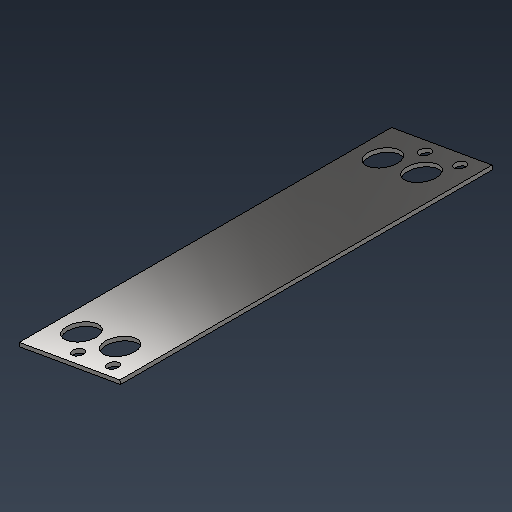
# Autodesk Inventor part: SteelFront
Saved by Autodesk Inventor 2026.2 (Build 302298010, 298A)
## iProperties
Created: 2026-04-07
Part Number: SteelFront
Material: Steel, Alloy
Document SubType Name: Modeling
Designer: szymo
Density: 7.73 g/cm^3
Appearance: Semi-Polished(2)
Mass: 19.4408 g
Surface Area: 54.2307 cm^2
Volume: 2.51498 cm^3
Author: szymo
Autodesk Inventor part; units mm, degrees
ref_plane "YZ Plane" through (0, 0, 0) normal (1, 0, 0) x (0, 1, 0)
ref_plane "XZ Plane" through (0, 0, 0) normal (0, 1, 0) x (-1, 0, 0)
ref_plane "XY Plane" through (0, 0, 0) normal (0, 0, 1) x (1, 0, 0)
sketch "Sketch1" plane through (0, 0, 0) normal (0, 0, 1) x (1, 0, 0)
  line L0 (0, -95.5) -> (0, -82.632) construction
  line L1 (2, -82.632) -> (2, -91.5) construction
  line L2 (2, -91.5) -> (4, -91.5) construction
  line L3 (4, -91.5) -> (0, -95.5) construction
  circle A0 centre (14.5, -55.2958) radius 14.5 construction
  line L4 (2.3736, -91.3) -> (29.4, -86.5356)
  line L5 (29.4, -86.5356) -> (29.2264, -85.5508)
  line L6 (29.2264, -85.5508) -> (2.2, -90.3152)
  line L7 (2.2, -90.3152) -> (2.3736, -91.3)
  line L8 (29.4, -86.5356) -> (29.4, -70.3377) construction
  line L9 (25, -86.2958) -> (4.5, -86.2958) projected
  line L10 (4.5, -86.2958) -> (4.5, -69.7958) projected
  line L11 (25, -69.7958) -> (4.5, -69.7958) projected
  line L12 (25, -86.2958) -> (25, -69.7958) projected
  line L13 (0, -82.632) -> (2, -82.632) projected
  dimension "d0" = 1
  dimension "d1" = 0.2
  dimension "d2" = 0.2
  dimension "d3" = 0.4
  dimension "d4" = 0
  constraints: 10 end point, 2 parallel, 1 perpendicular, 1 vertical
  measures "d0" distance between parallel lines of L6 L4
  measures "d1" distance from line of L1 L6.end
  measures "d2" distance from line of L2 L4.start
  measures "d3" distance edge to line of A0 L8
  measures "d4" distance from line of L6 L9.start
extrude "Extrusion1" add sketch "Sketch1" along normal mid plane 100 contours L7 L6 L5 L4
sketch "Sketch2" plane through (29.4, -86.5356, -50) normal (0.17361, -0.9848145, 0) x (0.9848145, 0.17361, 0)
  line L0 (-25.6154, 16.5) -> (-25.6154, 83.5) projected
  line L1 (-27.6462, 0) -> (-27.6462, 1) projected
  circle A0 centre (-5.2783, 96.6469) radius 1.5
  circle A1 centre (-14.8697, 96.6469) radius 1.5
  circle A2 centre (-14.8697, 3.3531) radius 1.5
  circle A3 centre (-5.2783, 3.3531) radius 1.5
  circle A4 centre (-9.5918, 90.5) radius 4
  circle A5 centre (-20.1476, 90.5) radius 4
  circle A6 centre (-9.5918, 9.5) radius 4
  circle A7 centre (-20.1476, 9.5) radius 4
  line L2 (-27.6462, 99) -> (-27.0065, 99) projected
  line L3 (-27.0065, 99) -> (-27.0065, 82.5) projected
  line L4 (-27.0065, 82.5) -> (-27.6462, 82.5) projected
  line L5 (-27.6462, 17.5) -> (-27.6462, 82.5) projected
  line L6 (-27.6462, 17.5) -> (-27.0065, 17.5) projected
  line L7 (-27.0065, 17.5) -> (-27.0065, 1) projected
  line L8 (-27.0065, 1) -> (-27.6462, 1) projected
  line L9 (-2.2607, 0) -> (-27.6462, 0) projected
  line L10 (-2.2607, 100) -> (-27.6462, 100) projected
  line L11 (-27.6462, 99) -> (-27.6462, 100) projected
  line L12 (-2.2607, 15.5) -> (-24.6, 15.5) projected
  ellipse E0 centre (-24.6, 16.5) end of major axis (-25.6154, 16.5) minor radius 1 (-25.6154, 16.5) -> (-24.6, 15.5) ccw projected
  ellipse E1 centre (-24.6, 83.5) end of major axis (-25.6154, 83.5) minor radius 1 (-24.6, 84.5) -> (-25.6154, 83.5) ccw projected
  line L13 (-2.2607, 84.5) -> (-24.6, 84.5) projected
  circle A8 centre (-14.9089, 96.6266) radius 2.25 projected
  circle A9 centre (-5.2607, 96.6266) radius 2.25 projected
  line L14 (-2.2607, 15.5) -> (-2.2607, 0) projected
  line L15 (-2.2607, 84.5) -> (-2.2607, 100) projected
  ellipse E2 centre (-20.2054, 90.5) end of major axis (-15.6612, 90.5) minor radius 4.5 (-16.268, 92.7467) -> (-16.268, 88.2533) ccw projected
  line L16 (-16.268, 92.7467) -> (-13.5497, 92.7467) projected
  ellipse E3 centre (-9.6123, 90.5) end of major axis (-5.0681, 90.5) minor radius 4.5 (-13.5497, 88.2533) -> (-13.5497, 92.7467) ccw projected
  line L17 (-13.5497, 88.2533) -> (-16.268, 88.2533) projected
  circle A10 centre (-14.9089, 3.3734) radius 2.25 projected
  circle A11 centre (-5.2607, 3.3734) radius 2.25 projected
  ellipse E4 centre (-20.2054, 9.5) end of major axis (-15.6612, 9.5) minor radius 4.5 (-16.268, 11.7467) -> (-16.268, 7.2533) ccw projected
  line L18 (-16.268, 11.7467) -> (-13.5497, 11.7467) projected
  ellipse E5 centre (-9.6123, 9.5) end of major axis (-5.0681, 9.5) minor radius 4.5 (-13.5497, 7.2533) -> (-13.5497, 11.7467) ccw projected
  line L19 (-13.5497, 7.2533) -> (-16.268, 7.2533) projected
  point P0 (-13.9301, 50)
  dimension "d7" = 3
  dimension "d8" = 3
  dimension "d9" = 3
  dimension "d10" = 3
  dimension "d13" = 8
  dimension "d14" = 8
  dimension "d15" = 8
  dimension "d16" = 8
  constraints: 8 centre point, 6 other
  measures "d7" diameter of A0
  measures "d8" diameter of A1
  measures "d9" diameter of A2
  measures "d10" diameter of A3
  measures "d13" diameter of A4
  measures "d14" diameter of A5
  measures "d15" diameter of A7
  measures "d16" diameter of A6
extrude "Extrusion2" cut sketch "Sketch2" against normal through all contours A0 | A1 | A2 | A3 | A4 | A5 | A6 | A7
equation "\"d14\" = d13"
equation "\"d15\" = d13"
equation "\"d16\" = d13"
body "Solid1"
